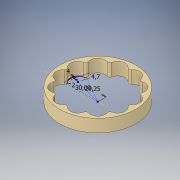
# Autodesk Inventor part: Enclosure
Saved by Autodesk Inventor 2018.3 (Build 223284000, 284)
## iProperties
Created: 2018-07-20
Part Number: Enclosure
Material: Generisch
Document SubType Name: Modeling
Designer: JochenAlt
Density: 1 g/cm^3
Appearance: Weizen
Author: JochenAlt
Autodesk Inventor part; units mm, degrees
ref_plane "YZ Plane" through (0, 0, 0) normal (1, 0, 0) x (0, 1, 0)
ref_plane "XZ Plane" through (0, 0, 0) normal (0, 1, 0) x (-1, 0, 0)
ref_plane "XY Plane" through (0, 0, 0) normal (0, 0, 1) x (1, 0, 0)
sketch "Skizze1" plane through (0, 0, 0) normal (0, 0, 1) x (1, 0, 0)
  line L0 (-46.7955, 0) -> (7.7993, 0) construction
  arc A0 (-28.7953, 16.625) -> (-33.25, 0) centre (0, 0) ccw
  arc A1 (-27.25, 0) -> (-27.9361, 1.5079) centre (-29.25, 0) ccw
  line L1 (0, 0) -> (-38.9963, 22.5145) construction
  line L2 (-29.25, 0) -> (0, 0) construction
  arc A2 (-24.9473, 12.6622) -> (-23.5992, 13.625) centre (-25.3312, 14.625) ccw
  arc A3 (-28.7665, 5.2962) -> (-29.25, 0) centre (0, 0) ccw construction
  arc A4 (-25.3312, 14.625) -> (-28.7665, 5.2962) centre (0, 0) ccw construction
  line L3 (-37.9513, 10.169) -> (0, 0) construction
  arc A5 (-24.9473, 12.6622) -> (-27.9361, 1.5079) centre (-23.7135, 6.354) ccw
  line L4 (-23.5992, 13.625) -> (-28.7953, 16.625)
  line L5 (-27.25, 0) -> (-33.25, 0)
  point P0 (-28.2533, 7.5705)
  dimension "d5" = 2
  dimension "d14" = 29.25
  dimension "d28" = 30
  dimension "d36" = 4.7
  dimension "d37" = 4
  constraints: 15 point on circle, 10 end point, 6 centre point, 6 point on line, 2 coincident, 2 collinear, 1 equal radius, 1 tangent, 1 other
  measures "d5" radius of A1
  measures "d14" distance of L1.start L2.start
  measures "d28" angle of L1 L0
  measures "d36" distance of point (-28.253, 7.57) A5.centre
  measures "d37" radial gap between concentric circles of A0 A4
extrude "Extrusion1" add sketch "Skizze1" along normal blind 11
pattern_circular "Runde Anordnung1" count 12 over 360 about axis through (0, 0, 0) along (0, 0, 1) of "Extrusion1"
